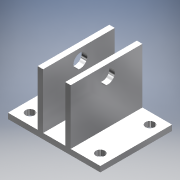
# Autodesk Inventor part: SDB 32
Saved by Autodesk Inventor 2019.4 (Build 234330000, 330)
## iProperties
Created: 2020-01-01
Part Number: SDB 32
Material: Stainless Steel
Document SubType Name: Modeling
Designer: Mark
Mass: 235.334 g
Surface Area: 168.784 cm^2
Volume: 29.4168 cm^3
Density: 8 g/cm^3
Appearance: Semi-Polished
Author: Mark
Autodesk Inventor part; units mm, degrees
ref_plane "YZ Plane" through (0, 0, 0) normal (1, 0, 0) x (0, 1, 0)
ref_plane "XZ Plane" through (0, 0, 0) normal (0, 1, 0) x (-1, 0, 0)
ref_plane "XY Plane" through (0, 0, 0) normal (0, 0, 1) x (1, 0, 0)
sketch "Sketch1" plane through (0, 0, 0) normal (0, 0, 1) x (1, 0, 0)
  line L0 (0, 0) -> (67, 0)
  line L1 (67, 0) -> (67, -4)
  line L2 (67, -4) -> (0, -4)
  line L3 (0, -4) -> (0, 0)
  dimension "d0" = 67
  dimension "d1" = 4
  constraints: 8 end point, 2 parallel, 1 horizontal, 1 perpendicular
  measures "d0" distance of L1.end L2.end
  measures "d1" distance of L0.end L1.end
extrude "Extrusion1" add sketch "Sketch1" along normal blind 52
sketch "Sketch2" plane through (0, 0, 0) normal (0, 1, 0) x (1, 0, 0)
  line L0 (8, -44) -> (59, -44)
  line L1 (59, -44) -> (59, -8)
  line L2 (59, -8) -> (8, -8)
  line L3 (8, -8) -> (8, -44)
  line L4 (8, -44) -> (59, -8) construction
  line L5 (59, -44) -> (8, -8) construction
  line L6 (0, 0) -> (0, -52) projected
  line L7 (0, 0) -> (67, 0) projected
  circle A0 centre (8, -8) radius 3.25
  circle A1 centre (59, -8) radius 3.25
  circle A2 centre (8, -44) radius 3.25
  circle A3 centre (59, -44) radius 3.25
  point P0 (33.5, -26)
  dimension "d4" = 51
  dimension "d5" = 36
  dimension "d6" = 8
  dimension "d7" = 8
  dimension "d8" = 6.5
  dimension "d9" = 6.5
  dimension "d10" = 6.5
  dimension "d11" = 6.5
  constraints: 12 end point, 4 centre point, 4 coincident, 2 midpoint, 2 parallel, 1 horizontal, 1 perpendicular
  measures "d4" distance of L2.end L1.end
  measures "d5" distance of L1.end L0.end
  measures "d6" distance between parallel lines of L6 L3
  measures "d7" distance between parallel lines of L7 L2
  measures "d8" diameter of A0
  measures "d9" diameter of A1
  measures "d10" diameter of A2
  measures "d11" diameter of A3
extrude "Extrusion2" cut sketch "Sketch2" against normal blind 4 contours L3 A2 L0 | L0 A2 L3 | A3 L1 L0 | L0 L1 A3 | A0 L2 L3 | L3 L2 A0 | A1 L2 L1 | L1 L2 A1
sketch "Sketch3" plane through (0, 0, 0) normal (0, 1, 0) x (1, 0, 0)
  line L0 (0, -52) -> (67, -52) projected
  line L1 (21.5, 0) -> (25.5, 0)
  line L2 (25.5, 0) -> (25.5, -52)
  line L3 (25.5, -52) -> (21.5, -52)
  line L4 (21.5, -52) -> (21.5, 0)
  line L5 (0, 0) -> (0, -52) projected
  line L6 (45.5, 0) -> (41.5, 0)
  line L7 (41.5, 0) -> (41.5, -52)
  line L8 (41.5, -52) -> (45.5, -52)
  line L9 (45.5, -52) -> (45.5, 0)
  line L10 (67, 0) -> (67, -52) projected
  dimension "d14" = 4
  dimension "d15" = 21.5
  dimension "d16" = 4
  dimension "d17" = 21.5
  dimension "d18" = 52
  dimension "d19" = 52
  constraints: 16 end point, 4 parallel, 2 horizontal, 2 perpendicular, 2 point on line
  measures "d14" distance of L2.end L3.end
  measures "d15" distance between parallel lines of L5 L4
  measures "d16" distance of L8.end L7.end
  measures "d17" distance between parallel lines of L10 L9
  measures "d18" distance of L8.end L6.start
  measures "d19" distance of L3.end L1.start
extrude "Extrusion3" add sketch "Sketch3" along normal blind 40
sketch "Sketch4" plane through (21.5, 0, 0) normal (-1, 0, 0) x (0, 0, 1)
  circle A0 centre (25, 32) radius 5
  line L0 (0, -4) -> (52, -4) projected
  line L1 (52, 0) -> (52, 40) projected
  point P0 (0, 0)
  dimension "d22" = 10
  dimension "d23" = 36
  dimension "d24" = 27
  constraints: 1 centre point
  measures "d22" diameter of A0
  measures "d23" distance from line of L0 A0.centre
  measures "d24" distance from line of L1 A0.centre
extrude "Extrusion4" cut sketch "Sketch4" against normal blind 40
body "Solid1"
